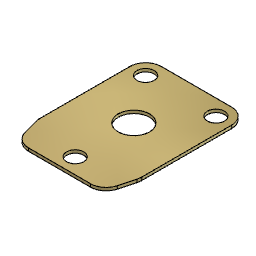
electorde puck v2 insulating plate CAM v4 (Autodesk Fusion 360 archive; units mm, degrees)
design "smb electrode top ground"
Autodesk Fusion 360 part; units mm, degrees
sketch "Sketch1" plane through (0, 0, 0) normal (0, 1, 0) x (1, 0, 0)
  circle A0 centre (-4.5, 13.5) radius 1.1
  circle A1 centre (4.5, 13.5) radius 1.1
  line L0 (0, -20) -> (0, -2.5) construction
  circle A2 centre (0, 0) radius 1.1
  circle A3 centre (0, 7.5) radius 2
  line L1 (-6.5, -2) -> (6.5, -2)
  line L2 (6.5, -2) -> (6.5, 15.5)
  line L3 (-6.5, -2) -> (-6.5, 15.5)
  line L4 (6.5, 15.5) -> (-6.5, 15.5)
  line L5 (-5.5, -2) -> (-6.5, 1.7321)
  line L6 (5.5, -2) -> (6.5, 1.7321)
  dimension "d1" = 2.2
  dimension "d2" = 2.2
  dimension "d3" = 9
  dimension "d4" = 13.5
  dimension "d5" = 2.2
  dimension "d6" = 7.5
  dimension "d7" = 4
  dimension "d8" = 13
  dimension "d9" = 2
  dimension "d10" = 2
  dimension "d15" = 30
  dimension "d16" = 11
  constraint horizontal A0.centre A1.centre
  constraint symmetric A0.centre A1.centre L0
  constraint coincident A2.centre origin
  constraint vertical A2.centre A3.centre
  constraint horizontal L1
  constraint perpendicular L1 L2
  constraint perpendicular L1 L3
  constraint perpendicular L2 L4
  constraint coincident L1 L5.start
  constraint coincident L3 L5.end
  constraint coincident L1 L6.start
  constraint coincident L2 L6.end
  constraint symmetric L0 L5 L6
  measures "d1" diameter of A0
  measures "d2" diameter of A1
  measures "d3" horizontal distance of A0.centre A1.centre
  measures "d4" vertical distance of A2.centre A1.centre
  measures "d5" diameter of A2
  measures "d6" distance of A2.centre A3.centre
  measures "d7" diameter of A3
  measures "d8" distance of L1.start L1.end
  measures "d9" distance of A2.centre L1
  measures "d10" distance of A1.centre L4
  measures "d15" angle of L5 L6
  measures "d16" distance of L5.start L6.start
extrude "Extrude1" add sketch "Sketch1" along normal blind 0.38 contours L1 L2 L3 L4 L5 L6
fillet "Fillet1" radius 2 6 edges at (-6.5, 0.19, -15.5) (6.5, 0.19, -15.5) (-5.5, 0.19, 2) (-6.5, 0.19, -1.7321) (5.5, 0.19, 2) (6.5, 0.19, -1.7321)

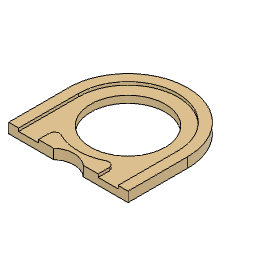
design "smb electrode insulators"
Autodesk Fusion 360 part; units mm, degrees
sketch "Sketch1" plane through (0, 0, 0) normal (0, 1, 0) x (1, 0, 0)
  line L0 (0, 0) -> (12, 0)
  line L1 (12, 0) -> (12, -12)
  line L2 (12, -12) -> (0, -12)
  line L3 (0, -12) -> (0, 0)
  circle A0 centre (6, -6) radius 3.75
  line L4 (6, 0) -> (6, -12) construction
  circle A1 centre (6, -6) radius 5
  line L5 (2, -12) -> (2, -9) construction
  line L6 (1, -12) -> (1, -6)
  line L7 (3, -10) -> (3, -12)
  arc A2 (7.5, -12) -> (4.5, -12) centre (6, -13.7) ccw
  dimension "d1" = 12
  dimension "d2" = 12
  dimension "d3" = 7.5
  dimension "d4" = 10
  dimension "d5" = 4
  dimension "d6" = 2
  dimension "d16" = 3
  dimension "d17" = 1.7
  constraint horizontal L0
  constraint vertical L1
  constraint horizontal L2
  constraint vertical L3
  constraint coincident L0.start L3.end
  constraint midpoint L0 L4.start
  constraint midpoint L2 L4.end
  constraint midpoint A0.centre L4
  constraint concentric A0 A1
  constraint coincident L2 L5.start
  constraint perpendicular L2 L5
  constraint coincident L2 L6.start
  constraint coincident A1 L6.end
  constraint perpendicular L2 L6
  constraint coincident A1 L7.start
  constraint coincident L2 L7.end
  constraint perpendicular L2 L7
  constraint coincident A1 L5.end
  constraint coincident L2 A2.start
  constraint coincident L2 A2.end
  constraint coincident L4 A2.centre
  measures "d1" distance of L0.start L2.end
  measures "d2" distance of L1.end L2.end
  measures "d3" diameter of A0
  measures "d4" diameter of A1
  measures "d5" distance of L4.end L5
  measures "d6" distance of L6 L7
  measures "d16" distance of A2.end A2.start
  measures "d17" distance of L2 A2.centre
extrude "Extrude1" add sketch "Sketch1" against normal blind 1 contours L0 L1 L2 L3 A1 L6 L7 A2 | L2 A1 L6 L7 | A1
extrude "Extrude2" cut sketch "Sketch1" against normal blind 0.3 contours A1
extrude "Extrude3" cut sketch "Sketch1" against normal blind 0.3 contours L2 A1 L6 L7
ref_plane "WorkPlane1" through (6, -0.5, 6) normal (1, 0, 0) x (0, 0, 1)
mirror "Mirror1" about plane through (6, -0.5, 6) normal (1, 0, 0) of "Extrude3"
fillet "Fillet1" radius 6 2 edges at (0, -0.5, 0) (12, -0.5, 0)
fillet "Fillet2" radius 0.5 2 edges at (3, -0.15, 10) (9, -0.15, 10)
equation "d3 = ( 3.75 * 2 ) * 1 mm"

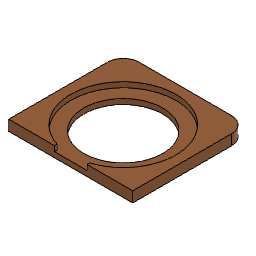
design "electrode puck v2 insulation"
Autodesk Fusion 360 part; units mm, degrees
sketch "Sketch1" plane through (0, 0, 0) normal (0, 1, 0) x (1, 0, 0)
  line L0 (0, 0) -> (12, 0)
  line L1 (12, 0) -> (12, -11)
  line L2 (12, -11) -> (0, -11)
  line L3 (0, -11) -> (0, 0)
  circle A0 centre (6, -6) radius 3.75
  line L4 (6, -11) -> (6, -6) construction
  line L5 (1, -11) -> (1, -1)
  line L6 (1, -1) -> (11, -1)
  line L7 (11, -1) -> (11, -11)
  circle A1 centre (6, -6) radius 5
  line L8 (4.45, -10.7537) -> (4.45, -11)
  line L9 (7.55, -10.7537) -> (7.55, -11)
  arc A2 (3.299, -11) -> (0.701, -11) centre (2, -11.75) ccw
  dimension "d1" = 12
  dimension "d2" = 11
  dimension "d3" = 5
  dimension "d4" = 7.5
  dimension "d5" = 1
  dimension "d11" = 10
  dimension "d12" = 3.1
  dimension "d14" = 1.5
  dimension "d15" = 4
  dimension "d16" = 0.75
  constraint horizontal L0
  constraint vertical L1
  constraint horizontal L2
  constraint vertical L3
  constraint coincident L0.start L3.end
  constraint midpoint L2 L4.start
  constraint coincident A0.centre L4.end
  constraint perpendicular L2 L4
  constraint concentric A0 A1
  constraint coincident A1 L8.start
  constraint coincident L2 L8.end
  constraint perpendicular L2 L8
  constraint coincident A1 L9.start
  constraint coincident L2 L9.end
  constraint perpendicular L2 L9
  constraint symmetric L4 L8 L9
  constraint coincident L2 A2.start
  constraint coincident L2 A2.end
  measures "d1" distance of L1.end L2.end
  measures "d2" distance of L0.end L1.end
  measures "d3" distance of L2 A0.centre
  measures "d4" diameter of A0
  measures "d11" diameter of A1
  measures "d12" distance of L8 L9
  measures "d14" radius of A2
  measures "d15" distance of L4 A2.centre
  measures "d16" distance of L2 A2.centre
extrude "Extrude1" add sketch "Sketch1" along normal blind 1 contours L0 L1 L2 L3 L5 L6 L7 A2 | L2 L5 A2 | L2 L7 A1 L9 | L2 L5 A2 | L2 L5 A1 L8 A2 | L6 L7 A1 | L5 L6 A1
extrude "Extrude2" add sketch "Sketch1" along normal blind 0.5 contours L2 L7 A1 L9 | L2 L5 A2 | L2 L5 A1 L8 A2 | L2 A1 L9 | L6 L7 A1 | A1 | L5 L6 A1 | L2 A1 L8 picked at (2.4911, -10.9389)
fillet "Fillet1" radius 1.5 2 edges at (12, 0.5, 0) (0, 0.5, 0)
move_face "OffsetFaces1" offset -0.1 3 faces at (12, 0.3333, 4.6667) (4.5, 0.3333, 0) (0, 0.3333, 7.8333)
